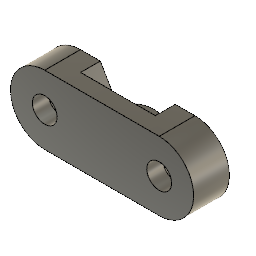
TOF_sensor_holder (Autodesk Fusion 360 design; units mm, degrees)
Autodesk Fusion 360 part; units mm, degrees
note: some values were not read from the file. Set by a fixed rule: which sketch regions a step uses; which face or edge a step refers to.
sketch "Sketch1" plane through (0, 0, 0) normal (0, 1, 0) x (1, 0, 0)
  line L0 (0, 0) -> (6.15, 0)
  circle A0 centre (7.148, 1.186) radius 1.55
  circle A1 centre (7.148, 1.186) radius 4.3
  line L1 (0, 0) -> (0, -3.114)
  line L2 (0, -3.114) -> (7.148, -3.114)
  line L3 (0, 0) -> (0, 5.486)
  line L4 (0, 5.486) -> (7.148, 5.486)
  dimension "d3" = 6.15
  dimension "d4" = 3.1
  dimension "d28" = 8.6
  constraint coincident L0.start L1.start
  constraint horizontal L0
  constraint coincident L0.end A0
  constraint concentric A0 A1
  constraint perpendicular L0 L1
  constraint coincident A1 L2.end
  constraint tangent A1 L2
  constraint perpendicular L1 L2
  constraint vertical L3
  constraint coincident A1 L4.end
  constraint tangent A1 L4
  constraint perpendicular L3 L4
  measures "d3" distance of L0.start L0.end
  measures "d4" diameter of A0
  measures "d28" diameter of A1
extrude "Extrude4" add sketch "Sketch1" along normal blind 2
sketch "Sketch5" plane through (0, 2, 0) normal (0, 1, 0) x (-1, 0, 0)
  circle A0 centre (-7.148, -1.186) radius 1.55
  line L0 (0, -5.486) -> (0, 3.114)
  line L1 (0, 3.114) -> (-7.148, 3.114)
  arc A1 (-7.148, 3.114) -> (-7.148, -5.486) centre (-7.148, -1.186) ccw
  line L2 (-7.148, -5.486) -> (0, -5.486)
  line L3 (-5.5285, -3.9843) -> (-3.9148, -1.1826)
  line L4 (-3.9148, -1.1826) -> (-5.5343, 1.6157)
  line L5 (-5.5343, 1.6157) -> (-8.7674, 1.6124)
  line L6 (-8.7674, 1.6124) -> (-10.3811, -1.1893)
  line L7 (-10.3811, -1.1893) -> (-8.7617, -3.9876)
  line L8 (-8.7617, -3.9876) -> (-5.5285, -3.9843)
  line L9 (-9.6345, 3.1118) -> (-12.1132, -1.1905)
  line L10 (-12.1132, -1.1905) -> (-9.6267, -5.4882)
  line L11 (-9.6267, -5.4882) -> (-4.6615, -5.4837)
  line L12 (-4.6615, -5.4837) -> (-2.1828, -1.1815)
  line L13 (-2.1828, -1.1815) -> (-4.6693, 3.1163)
  line L14 (-4.6693, 3.1163) -> (-9.6345, 3.1118)
  point P0 (-7.148, -1.186)
  point P1 (-7.148, -1.186)
  point P2 (-7.148, -1.186)
  point P3 (-7.148, -1.186)
  dimension "d38" = 2.8
  dimension "d39" = 4.3
  constraint coincident P2 P0
  constraint coincident P3 P0
  constraint coincident P3 P2
  measures "d38" distance of P3 L8
  measures "d39" distance of P3 L14
extrude "Extrude6" add sketch "Sketch5" along normal blind 2.48 contours L1 A1 L11 L12 L13
mirror "Mirror2" about plane through (0, 0, 0) normal (-1, 0, 0) of bodies 1 merged
sketch "Sketch6" plane through (0, 0, -5.486) normal (0, 0, -1) x (1, 0, 0)
  line L0 (7.148, 0) -> (-7.148, 0)
  line L1 (-7.148, -2) -> (-7.148, -4.48)
  line L2 (-7.148, -4.48) -> (-4.6615, -4.48)
  line L3 (-4.6615, -4.48) -> (-4.6615, -2)
  line L4 (-4.6615, -2) -> (-7.148, -2)
  line L5 (4.6615, -2) -> (4.6615, -4.48)
  line L6 (4.6615, -4.48) -> (7.148, -4.48)
  line L7 (7.148, -4.48) -> (7.148, -2)
  line L8 (0, 0) -> (0, -3.5)
  circle A0 centre (0, -3.5) radius 1.5
  circle A1 centre (0, -3.5) radius 3
  line L9 (7.148, -2) -> (4.6615, -2)
  line L10 (-7.148, 0) -> (-7.148, -2)
  line L11 (-7.148, -2) -> (7.148, -2)
  line L12 (7.148, -2) -> (7.148, 0)
  dimension "d42" = 3.5
  dimension "d43" = 3
  dimension "d44" = 6
  constraint coincident L8.start origin
  constraint perpendicular L0 L8
  constraint coincident L8.end A0.centre
  constraint concentric A0 A1
  measures "d42" distance of L8.start L8.end
  measures "d43" diameter of A0
  measures "d44" diameter of A1
extrude "Extrude7" add sketch "Sketch6" against normal blind 4.72 contours A1 L11
extrude "Extrude8" add 2 faces at (3.2859, 2, -4.2899) (-3.2859, 2, -4.2907) along direction (0, 1, 0) up to surface end surface through (0, 4.48, 0) normal (0, 1, 0) offset 0
fillet "Fillet2" radius 0.5 12 edges at (7.1509, 4.48, 1.614) (9.5743, 4.48, 0.2115) (9.5714, 4.48, -2.5885) (7.1451, 4.48, -3.986) (4.7217, 4.48, -2.5835) (4.7246, 4.48, 0.2165) (-7.1509, 4.48, 1.614) (-4.7246, 4.48, 0.2165) (-4.7217, 4.48, -2.5835) (-7.1451, 4.48, -3.986) (-9.5714, 4.48, -2.5885) (-9.5743, 4.48, 0.2115)
equation "hole_diameter = 3.1 mm"
equation "hole_edge2edge = 12.3 mm"
equation "d3 = hole_edge2edge / 2"
equation "d4 = hole_diameter"
equation "d28 = 5.6 mm + 1.5 mm * 2"
equation "tabWidth = 2 mm"
equation "d38 = ( 5.6 / 2 ) * 1 mm"
equation "d39 = ( 5.6 / 2 ) * 1 mm + 1.5 mm"
equation "d42 = 3 mm / 2 + 2 mm"
equation "d44 = 3 mm + 3 mm"
equation "d45 = -( ( 5.44 / 2 ) * 1 mm + 2 mm )"
